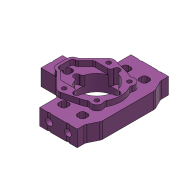
# Autodesk Inventor part: 16_030_TIBIA_SENSOR_BASE_R1
Saved by Autodesk Inventor 2021.2 (Build 252289000, 289)
## iProperties
Created: 2018-07-25
Part Number: 16_030_TIBIA_SENSOR_BASE_R1
Material: ABS プラスチック
Document SubType Name: Modeling
Designer: y6tada
Density: 1.06 g/cm^3
Appearance: 滑らか - 紫
Mass: 3.15209 g
Surface Area: 27.7865 cm^2
Volume: 2.97367 cm^3
Author: y6tada
Autodesk Inventor part; units mm, degrees
ref_plane "YZ Plane" through (0, 0, 0) normal (1, 0, 0) x (0, 1, 0)
ref_plane "XZ Plane" through (0, 0, 0) normal (0, 1, 0) x (-1, 0, 0)
ref_plane "作業平面1" through (0, 0, 0) normal (0, 0, 1) x (1, 0, 0)
sketch "スケッチ1" plane through (0, 0, 0) normal (0, 0, 1) x (1, 0, 0)
  line L0 (0, 0) -> (12.25, 0)
  line L1 (12.25, 0) -> (12.25, 14.0352) construction
  line L2 (-1.75, 17) -> (-1.75, 11.1093)
  line L3 (-2.0429, 10.4022) -> (-8.1522, 4.2929)
  line L4 (-8.8593, 4) -> (-14.25, 4)
  line L5 (-14.25, 4) -> (-14.25, 0.6)
  line L6 (-14.05, 0) -> (0, 0)
  line L7 (-8.7985, 4.3535) -> (-8.4451, 4) construction
  arc A0 (-8.8593, 4) -> (-8.1522, 4.2929) centre (-8.8593, 5) ccw
  arc A1 (-2.0429, 10.4022) -> (-1.75, 11.1093) centre (-2.75, 11.1093) ccw
  arc A2 (1.15, 17) -> (2.35, 17) centre (1.75, 17.8) ccw
  arc A3 (8.15, 17) -> (9.35, 17) centre (8.75, 17.8) ccw
  line L8 (12.25, 17) -> (9.35, 17)
  line L9 (8.15, 17) -> (2.35, 17)
  line L10 (1.15, 17) -> (-1.75, 17)
  line L11 (8.75, 17.8) -> (1.75, 17.8) construction
  arc A4 (-14.05, 0) -> (-14.25, 0.6) centre (-15.05, 0) ccw
  line L12 (12.455, 13.618) -> (14.045, 10.382)
  line L13 (14.25, 9.5) -> (14.25, 0)
  line L14 (14.25, 0) -> (12.25, 0)
  line L15 (12.25, 14.5) -> (12.25, 17)
  arc A5 (12.25, 14.5) -> (12.455, 13.618) centre (14.25, 14.5) ccw
  arc A6 (14.25, 9.5) -> (14.045, 10.382) centre (12.25, 9.5) ccw
  dimension "d5" = 1
  dimension "d9" = 1
  dimension "d21" = 14.25
  dimension "d22" = 4
  dimension "d23" = 8.8
  dimension "d24" = 45
  dimension "d26" = 17
  dimension "d27" = 0.8
  dimension "d28" = 1
  dimension "d29" = 3.5
  dimension "d30" = 3.5
  dimension "d31" = 1
  dimension "d32" = 0.8
  dimension "d73" = 1.75
  dimension "d74" = 14.25
  dimension "d76" = 14
  dimension "d77" = 2
  dimension "d78" = 2.5
  dimension "d79" = 5
  constraints: 32 end point, 14 point on circle, 8 tangent, 7 centre point, 6 horizontal, 5 point on line, 5 vertical, 3 perpendicular, 2 collinear, 2 equal radius, 1 coincident, 2 other
  measures "d5" radius of A0
  measures "d9" radius of A1
  measures "d21" distance from line of L5 point (0, 0)
  measures "d22" distance between parallel lines of L6 L4
  measures "d23" distance from line of L0.start L3
  measures "d24" angle of L3 L6
  measures "d26" distance of L0.end L8.start
  measures "d27" distance between parallel lines of L11 L9
  measures "d28" radius of A3
  measures "d29" distance from line of L11.start L1
  measures "d30" distance from line of L11.end L2
  measures "d31" radius of A4
  measures "d32" distance from line of L5 A4.centre
  measures "d73" distance from line of L0.start L2
  measures "d74" distance from line of L0.start L13
  measures "d76" distance between parallel lines of L2 L15
  measures "d77" radius of A5
  measures "d78" distance from line of A5.centre L8
  measures "d79" vertical distance of A6.centre A5.centre
extrude "押し出し1" add sketch "スケッチ1" along normal blind 6
sketch "スケッチ3" plane through (2.35, 17, 0) normal (0, 1, 0) x (1, 0, 0)
  circle A0 centre (-0.6, -3) radius 1.25
  circle A1 centre (6.4, -3) radius 1.25
  line L0 (6.4, -3) -> (-0.6, -3) construction
  line L1 (6.4, -3) -> (6.4, 0) construction
  line L2 (7, 0) -> (5.8, 0) construction
  line L3 (-0.6, -3) -> (-0.6, 0) construction
  line L4 (0, 0) -> (-1.2, 0) construction
  point P0 (-2.35, 0)
  dimension "d33" = 3
  dimension "d34" = 2.5
  constraints: 6 end point, 2 centre point, 2 midpoint, 2 vertical, 1 equal radius, 1 horizontal
  measures "d33" distance from line of point (-2.35, 0) L0
  measures "d34" diameter of A0
extrude "押し出し3" cut sketch "スケッチ3" against normal blind 5
mirror "ミラー2" about plane through (0, 0, 0) normal (0, -1, 0) of "押し出し1", "押し出し3"
sketch "スケッチ4" plane through (-14.25, -4, 0) normal (-1, 0, 0) x (0, 0, 1)
  circle A0 centre (3, 4) radius 1.25
  line L0 (0, 4) -> (3, 4) construction
  dimension "d37" = 3
  dimension "d38" = 2.5
  constraints: 2 end point, 1 centre point, 1 horizontal
  measures "d37" distance of L0.start L0.end
  measures "d38" diameter of A0
extrude "押し出し4" cut sketch "スケッチ4" against normal blind 5
sketch "スケッチ5" plane through (0, 0, 6) normal (0, 0, 1) x (1, 0, 0)
  circle A0 centre (2.5456, 0) radius 6.6
  line L0 (0, 0) -> (2.5456, 0) construction
  line L1 (-2.0429, 10.4022) -> (-8.1522, 4.2929) construction
  line L2 (0.7855, 7.5738) -> (-6.3238, 0.4645) construction
  dimension "d41" = 13.2
  dimension "d59" = 4
  constraints: 4 end point, 1 centre point, 1 coincident, 1 horizontal, 1 parallel, 1 tangent, 1 other
  measures "d41" diameter of A0
  measures "d59" distance between parallel lines of L2 L1
extrude "押し出し5" cut sketch "スケッチ5" against normal blind 8
sketch "スケッチ6" plane through (0, 0, 6) normal (0, 0, 1) x (1, 0, 0)
  line L0 (-4.9544, 0) -> (2.5456, 0) construction
  line L1 (-4.9544, 1.1) -> (-4.8334, 1.1)
  line L2 (-4.9544, -1.1) -> (-4.8334, -1.1)
  circle A0 centre (2.5456, 0) radius 6.6 construction
  arc A1 (-4.9544, 1.1) -> (-4.9544, -1.1) centre (-4.9544, 0) ccw
  arc A2 (-3.7793, -1.8857) -> (-4.8334, -1.1) centre (-4.8334, -2.2) ccw
  arc A3 (-4.8334, 1.1) -> (-3.7793, 1.8857) centre (-4.8334, 2.2) ccw
  arc A4 (-3.7793, 1.8857) -> (-3.7793, -1.8857) centre (2.5456, 0) ccw
  point P0 (-2.4621, -1.1)
  point P1 (-2.4621, 1.1)
  dimension "d76" = 14
  dimension "d44" = 7.5
  dimension "d47" = 1.1
  dimension "d53" = 1.1
  dimension "d55" = 1.1
  constraints: 8 point on circle, 6 end point, 6 tangent, 4 centre point, 3 horizontal, 2 concentric, 2 point on line, 1 coincident
  measures "d44" distance of L0.start L0.end
  measures "d47" radius of A1
  measures "d53" radius of A2
  measures "d55" radius of A3
extrude "押し出し6" cut sketch "スケッチ6" against normal blind 3.5
pattern_circular "円形状パターン1" count 4 over 360 about axis through (2.5456, 0, 6) along (0, 0, -1) of "押し出し6"
sketch "スケッチ9" plane through (0, 0, 6) normal (0, 0, 1) x (1, 0, 0)
  arc A0 (1.4456, -7.379) -> (0.6599, -6.3249) centre (0.3456, -7.379) ccw
  arc A1 (10.0456, -1.1) -> (11.1456, 0) centre (10.0456, 0) ccw
  line L0 (10.0456, -1.1) -> (9.9246, -1.1)
  arc A2 (9.9246, -1.1) -> (8.8705, -1.8857) centre (9.9246, -2.2) ccw
  arc A3 (4.4313, -6.3249) -> (8.8705, -1.8857) centre (2.5456, 0) ccw
  arc A4 (4.4313, -6.3249) -> (3.6456, -7.379) centre (4.7456, -7.379) ccw
  line L1 (3.6456, -7.379) -> (3.6456, -7.5)
  arc A5 (1.4456, -7.5) -> (3.6456, -7.5) centre (2.5456, -7.5) ccw
  line L2 (1.4456, -7.5) -> (1.4456, -7.379)
  arc A6 (10.4511, -4.3014) -> (11.5456, 0) centre (2.5456, 0) ccw
  arc A7 (7.7588, -7.883) -> (10.4286, -5.2133) centre (8.6267, -6.0811) ccw
  arc A8 (4.863, -8.6965) -> (6.847, -7.9056) centre (2.5456, 0) ccw
  arc A9 (10.4511, -4.3014) -> (10.4286, -5.2133) centre (11.3295, -4.7793) ccw
  arc A10 (7.7588, -7.883) -> (6.847, -7.9056) centre (7.3249, -8.784) ccw
  line L3 (-8.1522, -4.2929) -> (-2.7518, -9.6932)
  line L4 (-2.0429, -10.4022) -> (-8.1522, -4.2929) construction
  arc A11 (1.4456, -7.379) -> (0.6599, -6.3249) centre (0.3456, -7.379) ccw projected
  line L5 (-4.7518, -6.279) -> (-7.738, -3.2929)
  line L6 (-9.4544, -2) -> (-9.4544, 0)
  arc A12 (1.4456, -7.379) -> (0.3456, -6.279) centre (0.3456, -7.379) ccw
  line L7 (0.3456, -6.279) -> (-4.7518, -6.279)
  line L8 (2.5456, 0) -> (-9.4544, 0) construction
  line L9 (2.5456, 7.5) -> (2.5456, 0) construction
  line L10 (2.5456, 0) -> (10.0456, 0) construction
  line L11 (2.5456, 0) -> (2.5456, -7.5) construction
  line L12 (-2.0429, -10.4022) -> (-8.1522, -4.2929) construction
  circle A13 centre (2.5456, 0) radius 2.8146 construction
  arc A14 (-2.7518, -9.6932) -> (-0.8227, -10.2116) centre (-1.3376, -8.279) ccw
  line L13 (-0.8227, -10.2116) -> (4.863, -8.6965)
  line L14 (-10.4544, 0) -> (-9.4544, 0)
  line L15 (-10.4544, 0) -> (-10.4544, -2)
  line L16 (10.0456, 0) -> (11.1456, 0) construction
  line L17 (11.1456, 0) -> (11.5456, 0)
  line L18 (8.6267, -6.0811) -> (2.5456, 0) construction
  line L19 (-8.8593, -4) -> (-14.25, -4) construction
  arc A15 (-10.4544, -2) -> (-8.9846, -3.9284) centre (-8.4544, -2) ccw
  arc A16 (-8.1522, -4.2929) -> (-8.8593, -4) centre (-8.8593, -5) ccw construction
  arc A17 (-8.1522, -4.2929) -> (-8.5942, -4.0358) centre (-8.8593, -5) ccw
  line L20 (-8.4544, -3) -> (-8.4451, -3)
  arc A18 (-9.4544, -2) -> (-8.4544, -3) centre (-8.4544, -2) ccw
  arc A19 (-7.738, -3.2929) -> (-8.4451, -3) centre (-8.4451, -4) ccw
  line L21 (-8.9846, -3.9284) -> (-8.5942, -4.0358)
  point P0 (-10.4544, -1.5765)
  point P1 (-9.4544, -1.5765)
  point P2 (-10.05, -4)
  dimension "d80" = 1.1
  dimension "d84" = 7.5
  dimension "d86" = 1.1
  dimension "d87" = 1.1
  dimension "d91" = 2
  dimension "d92" = 2
  dimension "d93" = 12
  dimension "d94" = 9
  dimension "d95" = 2
  dimension "d96" = 8.6
  dimension "d97" = 45
  dimension "d98" = 1
  dimension "d113" = 1
  dimension "d114" = 1
  dimension "d115" = 1
  dimension "d116" = 1
  dimension "d117" = 1
  constraints: 38 end point, 32 point on circle, 23 centre point, 14 tangent, 5 point on line, 4 concentric, 4 horizontal, 4 vertical, 3 collinear, 2 equal radius, 2 perpendicular, 1 coincident, 1 parallel, 7 other
  measures "d80" radius of A0
  measures "d84" distance of L8.start L10.end
  measures "d86" radius of A5
  measures "d87" radius of A4
  measures "d91" radius of A14
  measures "d92" distance from line of L7 A14.centre
  measures "d93" distance between parallel lines of L11 L6
  measures "d94" radius of A8
  measures "d95" radius of A7
  measures "d96" distance of L18.start L18.end
  measures "d97" angle of L8 L18
  measures "d98" radius of A10
  measures "d113" distance between parallel lines of L15 L6
  measures "d114" distance between parallel lines of L3 L5
  measures "d115" radius of A18
  measures "d116" radius of A19
  measures "d117" distance between parallel lines of L19 L20
extrude "押し出し7" add sketch "スケッチ9" along normal blind 2
mirror "ミラー3" about plane through (0, 0, 0) normal (0, 1, 0) of "押し出し7"
fillet "フィレット1" radius 1 2 edges at (-4.7518, -6.279, 7) (-4.7518, 6.279, 7)
sketch "スケッチ10" plane through (0, 0, 6) normal (0, 0, 1) x (1, 0, 0)
  line L0 (-9.4544, -2) -> (-9.4544, 2) construction
  line L1 (-8.4544, 1.5) -> (-7.9544, 1.5)
  line L2 (-6.9544, 0.5) -> (-6.9544, -0.5)
  line L3 (-7.9544, -1.5) -> (-8.4544, -1.5)
  line L4 (-9.4544, -0.5) -> (-9.4544, 0.5)
  arc A0 (-8.4544, 1.5) -> (-9.4544, 0.5) centre (-8.4544, 0.5) ccw
  arc A1 (-6.9544, 0.5) -> (-7.9544, 1.5) centre (-7.9544, 0.5) ccw
  arc A2 (-7.9544, -1.5) -> (-6.9544, -0.5) centre (-7.9544, -0.5) ccw
  arc A3 (-9.4544, -0.5) -> (-8.4544, -1.5) centre (-8.4544, -0.5) ccw
  line L5 (-0.0673, 0) -> (5.25, 0) construction
  line L6 (1.25, -10) -> (2.25, -10)
  line L7 (3.25, -11) -> (3.25, -12)
  line L8 (2.25, -13) -> (1.25, -13)
  line L9 (0.25, -12) -> (0.25, -11)
  arc A4 (1.25, -10) -> (0.25, -11) centre (1.25, -11) ccw
  arc A5 (3.25, -11) -> (2.25, -10) centre (2.25, -11) ccw
  arc A6 (2.25, -13) -> (3.25, -12) centre (2.25, -12) ccw
  arc A7 (0.25, -12) -> (1.25, -13) centre (1.25, -12) ccw
  arc A8 (2.35, -17) -> (1.15, -17) centre (1.75, -17.8) ccw construction
  arc A9 (9.35, -17) -> (8.15, -17) centre (8.75, -17.8) ccw construction
  line L10 (1.75, -17.8) -> (8.75, -17.8) construction
  line L11 (5.25, -17.8) -> (5.25, -9.3652) construction
  line L12 (1.75, -13) -> (1.75, -10) construction
  line L13 (8.15, -17) -> (2.35, -17) projected
  line L14 (9.25, -10) -> (8.25, -10)
  line L15 (7.25, -11) -> (7.25, -12)
  line L16 (8.25, -13) -> (9.25, -13)
  line L17 (10.25, -12) -> (10.25, -11)
  arc A10 (10.25, -11) -> (9.25, -10) centre (9.25, -11) ccw
  arc A11 (8.25, -10) -> (7.25, -11) centre (8.25, -11) ccw
  arc A12 (7.25, -12) -> (8.25, -13) centre (8.25, -12) ccw
  arc A13 (9.25, -13) -> (10.25, -12) centre (9.25, -12) ccw
  line L18 (8.75, -13) -> (8.75, -10) construction
  line L19 (1.25, 10) -> (2.25, 10)
  line L20 (3.25, 11) -> (3.25, 12)
  line L21 (2.25, 13) -> (1.25, 13)
  line L22 (0.25, 12) -> (0.25, 11)
  arc A14 (0.25, 11) -> (1.25, 10) centre (1.25, 11) ccw
  arc A15 (2.25, 10) -> (3.25, 11) centre (2.25, 11) ccw
  arc A16 (3.25, 12) -> (2.25, 13) centre (2.25, 12) ccw
  arc A17 (1.25, 13) -> (0.25, 12) centre (1.25, 12) ccw
  line L23 (1.75, 13) -> (1.75, 10) construction
  line L24 (9.25, 10) -> (8.25, 10)
  arc A18 (9.25, 10) -> (10.25, 11) centre (9.25, 11) ccw
  line L25 (10.25, 12) -> (10.25, 11)
  arc A19 (7.25, 11) -> (8.25, 10) centre (8.25, 11) ccw
  arc A20 (10.25, 12) -> (9.25, 13) centre (9.25, 12) ccw
  line L26 (7.25, 11) -> (7.25, 12)
  line L27 (8.75, 13) -> (8.75, 10) construction
  line L28 (8.25, 13) -> (9.25, 13)
  arc A21 (8.25, 13) -> (7.25, 12) centre (8.25, 12) ccw
  line L29 (-9.4544, 2) -> (-9.4544, -2) projected
  point P0 (0, 0)
  dimension "d103" = 1
  dimension "d104" = 2.5
  dimension "d105" = 1
  dimension "d106" = 1
  dimension "d107" = 3
  dimension "d108" = 3
  dimension "d109" = 4
  dimension "d118" = 1
  constraints: 54 end point, 42 symmetric about line, 40 point on circle, 20 centre point, 16 tangent, 5 equal radius, 4 horizontal, 4 parallel, 3 midpoint, 2 perpendicular, 2 point on line, 1 collinear, 1 vertical, 14 other
  measures "d103" radius of A0
  measures "d104" distance between parallel lines of L0 L2
  measures "d105" radius of A4
  measures "d106" radius of A5
  measures "d107" distance between parallel lines of L7 L9
  measures "d108" distance between parallel lines of L8 L6
  measures "d109" distance between parallel lines of L13 L8
  measures "d118" distance of A1.centre A2.centre
extrude "押し出し8" cut sketch "スケッチ10" against normal blind 6
sketch "スケッチ11" plane through (0, 0, 8) normal (0, 0, 1) x (1, 0, 0)
  arc A0 (-0.8227, 10.2116) -> (-2.7518, 9.6932) centre (-1.3376, 8.279) ccw projected
  circle A1 centre (-1.3376, 8.279) radius 0.8
  circle A2 centre (8.6267, 6.0811) radius 0.8
  circle A3 centre (8.6267, -6.0811) radius 0.8
  circle A4 centre (-1.3376, -8.279) radius 0.8
  arc A5 (-0.8227, 10.2116) -> (-2.7518, 9.6932) centre (-1.3376, 8.279) ccw projected
  arc A6 (10.4286, 5.2133) -> (7.7588, 7.883) centre (8.6267, 6.0811) ccw projected
  arc A7 (7.7588, -7.883) -> (10.4286, -5.2133) centre (8.6267, -6.0811) ccw projected
  arc A8 (-2.7518, -9.6932) -> (-0.8227, -10.2116) centre (-1.3376, -8.279) ccw projected
  point P0 (0, 0)
  dimension "d119" = 1.6
  constraints: 4 centre point, 4 concentric, 3 equal radius, 1 coincident
  measures "d119" diameter of A1
extrude "押し出し9" cut sketch "スケッチ11" against normal blind 8
sketch "スケッチ12" plane through (0, 0, 8) normal (0, 0, 1) x (1, 0, 0)
  circle A0 centre (8.6267, -6.0811) radius 0.8 projected
  circle A1 centre (-1.3376, 8.279) radius 0.8 projected
  circle A2 centre (8.6267, 6.0811) radius 0.8 projected
  circle A3 centre (-1.3376, -8.279) radius 0.8 projected
  arc A4 (10.0456, -1.1) -> (10.0456, 1.1) centre (10.0456, 0) ccw projected
  line L0 (10.0456, -1.1) -> (9.9246, -1.1) projected
  arc A5 (9.9246, -1.1) -> (8.8705, -1.8857) centre (9.9246, -2.2) ccw projected
  arc A6 (4.4313, -6.3249) -> (8.8705, -1.8857) centre (2.5456, 0) ccw projected
  arc A7 (4.4313, -6.3249) -> (3.6456, -7.379) centre (4.7456, -7.379) ccw projected
  line L1 (3.6456, -7.379) -> (3.6456, -7.5) projected
  arc A8 (1.4456, -7.5) -> (3.6456, -7.5) centre (2.5456, -7.5) ccw projected
  line L2 (1.4456, -7.5) -> (1.4456, -7.379) projected
  arc A9 (1.4456, -7.379) -> (0.3456, -6.279) centre (0.3456, -7.379) ccw projected
  line L3 (0.3456, -6.279) -> (-4.3376, -6.279) projected
  arc A10 (-5.0447, -5.9861) -> (-4.3376, -6.279) centre (-4.3376, -5.279) ccw projected
  line L4 (-5.0447, -5.9861) -> (-7.738, -3.2929) projected
  arc A11 (-7.738, -3.2929) -> (-8.4451, -3) centre (-8.4451, -4) ccw projected
  line L5 (-8.4451, -3) -> (-8.4544, -3) projected
  arc A12 (-9.4544, -2) -> (-8.4544, -3) centre (-8.4544, -2) ccw projected
  line L6 (-9.4544, -2) -> (-9.4544, 2) projected
  arc A13 (-8.4544, 3) -> (-9.4544, 2) centre (-8.4544, 2) ccw projected
  line L7 (-8.4451, 3) -> (-8.4544, 3) projected
  arc A14 (-8.4451, 3) -> (-7.738, 3.2929) centre (-8.4451, 4) ccw projected
  line L8 (-5.0447, 5.9861) -> (-7.738, 3.2929) projected
  arc A15 (-4.3376, 6.279) -> (-5.0447, 5.9861) centre (-4.3376, 5.279) ccw projected
  line L9 (0.3456, 6.279) -> (-4.3376, 6.279) projected
  arc A16 (0.3456, 6.279) -> (1.4456, 7.379) centre (0.3456, 7.379) ccw projected
  line L10 (1.4456, 7.5) -> (1.4456, 7.379) projected
  arc A17 (3.6456, 7.5) -> (1.4456, 7.5) centre (2.5456, 7.5) ccw projected
  line L11 (3.6456, 7.379) -> (3.6456, 7.5) projected
  arc A18 (3.6456, 7.379) -> (4.4313, 6.3249) centre (4.7456, 7.379) ccw projected
  arc A19 (8.8705, 1.8857) -> (4.4313, 6.3249) centre (2.5456, 0) ccw projected
  arc A20 (8.8705, 1.8857) -> (9.9246, 1.1) centre (9.9246, 2.2) ccw projected
  line L12 (10.0456, 1.1) -> (9.9246, 1.1) projected
  arc A21 (10.4511, -4.3014) -> (10.4511, 4.3014) centre (2.5456, 0) ccw projected
  arc A22 (10.4286, 5.2133) -> (10.4511, 4.3014) centre (11.3295, 4.7793) ccw projected
  arc A23 (10.4286, 5.2133) -> (7.7588, 7.883) centre (8.6267, 6.0811) ccw projected
  arc A24 (6.847, 7.9056) -> (7.7588, 7.883) centre (7.3249, 8.784) ccw projected
  arc A25 (6.847, 7.9056) -> (4.863, 8.6965) centre (2.5456, 0) ccw projected
  line L13 (-0.8227, 10.2116) -> (4.863, 8.6965) projected
  arc A26 (-0.8227, 10.2116) -> (-2.7518, 9.6932) centre (-1.3376, 8.279) ccw projected
  line L14 (-8.1522, 4.2929) -> (-2.7518, 9.6932) projected
  arc A27 (-8.5942, 4.0358) -> (-8.1522, 4.2929) centre (-8.8593, 5) ccw projected
  line L15 (-8.9846, 3.9284) -> (-8.5942, 4.0358) projected
  arc A28 (-8.9846, 3.9284) -> (-10.4544, 2) centre (-8.4544, 2) ccw projected
  line L16 (-10.4544, -2) -> (-10.4544, 2) projected
  arc A29 (-10.4544, -2) -> (-8.9846, -3.9284) centre (-8.4544, -2) ccw projected
  line L17 (-8.9846, -3.9284) -> (-8.5942, -4.0358) projected
  arc A30 (-8.1522, -4.2929) -> (-8.5942, -4.0358) centre (-8.8593, -5) ccw projected
  line L18 (-8.1522, -4.2929) -> (-2.7518, -9.6932) projected
  arc A31 (-2.7518, -9.6932) -> (-0.8227, -10.2116) centre (-1.3376, -8.279) ccw projected
  line L19 (-0.8227, -10.2116) -> (4.863, -8.6965) projected
  arc A32 (4.863, -8.6965) -> (6.847, -7.9056) centre (2.5456, 0) ccw projected
  arc A33 (7.7588, -7.883) -> (6.847, -7.9056) centre (7.3249, -8.784) ccw projected
  arc A34 (7.7588, -7.883) -> (10.4286, -5.2133) centre (8.6267, -6.0811) ccw projected
  arc A35 (10.4511, -4.3014) -> (10.4286, -5.2133) centre (11.3295, -4.7793) ccw projected
  line L20 (-4.9544, 1.1) -> (-4.8334, 1.1) projected
  arc A36 (-4.9544, 1.1) -> (-4.9544, -1.1) centre (-4.9544, 0) ccw projected
  line L21 (-4.8334, -1.1) -> (-4.9544, -1.1) projected
  arc A37 (-3.7793, -1.8857) -> (-4.8334, -1.1) centre (-4.8334, -2.2) ccw projected
  arc A38 (-3.7793, 1.8857) -> (-3.7793, -1.8857) centre (2.5456, 0) ccw projected
  arc A39 (-4.8334, 1.1) -> (-3.7793, 1.8857) centre (-4.8334, 2.2) ccw projected
  arc A40 (0.6599, 6.3249) -> (-3.7793, 1.8857) centre (2.5456, 0) ccw projected
  arc A41 (-3.7793, -1.8857) -> (0.6599, -6.3249) centre (2.5456, 0) ccw projected
  arc A42 (-9.4544, -0.5) -> (-8.4544, -1.5) centre (-8.4544, -0.5) ccw projected
  line L22 (-9.4544, -0.5) -> (-9.4544, -2) projected
  arc A43 (-9.4544, -2) -> (-8.4544, -3) centre (-8.4544, -2) ccw projected
  line L23 (-8.4544, -3) -> (-8.4451, -3) projected
  arc A44 (-7.738, -3.2929) -> (-8.4451, -3) centre (-8.4451, -4) ccw projected
  line L24 (-7.738, -3.2929) -> (-5.0447, -5.9861) projected
  arc A45 (-5.0447, -5.9861) -> (-4.3376, -6.279) centre (-4.3376, -5.279) ccw projected
  line L25 (-4.3376, -6.279) -> (0.3456, -6.279) projected
  arc A46 (0.6599, -6.3249) -> (0.3456, -6.279) centre (0.3456, -7.379) ccw projected
  arc A47 (-3.7793, -1.8857) -> (0.6599, -6.3249) centre (2.5456, 0) ccw projected
  arc A48 (-3.7793, -1.8857) -> (-4.8334, -1.1) centre (-4.8334, -2.2) ccw projected
  line L26 (-4.8334, -1.1) -> (-4.9544, -1.1) projected
  arc A49 (-4.9544, 1.1) -> (-4.9544, -1.1) centre (-4.9544, 0) ccw projected
  line L27 (-4.9544, 1.1) -> (-4.8334, 1.1) projected
  arc A50 (-4.8334, 1.1) -> (-3.7793, 1.8857) centre (-4.8334, 2.2) ccw projected
  arc A51 (0.6599, 6.3249) -> (-3.7793, 1.8857) centre (2.5456, 0) ccw projected
  arc A52 (0.3456, 6.279) -> (0.6599, 6.3249) centre (0.3456, 7.379) ccw projected
  line L28 (0.3456, 6.279) -> (-4.3376, 6.279) projected
  arc A53 (-4.3376, 6.279) -> (-5.0447, 5.9861) centre (-4.3376, 5.279) ccw projected
  line L29 (-5.0447, 5.9861) -> (-7.738, 3.2929) projected
  arc A54 (-8.4451, 3) -> (-7.738, 3.2929) centre (-8.4451, 4) ccw projected
  line L30 (-8.4451, 3) -> (-8.4544, 3) projected
  arc A55 (-8.4544, 3) -> (-9.4544, 2) centre (-8.4544, 2) ccw projected
  line L31 (-9.4544, 2) -> (-9.4544, 0.5) projected
  arc A56 (-8.4544, 1.5) -> (-9.4544, 0.5) centre (-8.4544, 0.5) ccw projected
  line L32 (-8.4544, 1.5) -> (-7.9544, 1.5) projected
  arc A57 (-6.9544, 0.5) -> (-7.9544, 1.5) centre (-7.9544, 0.5) ccw projected
  line L33 (-6.9544, 0.5) -> (-6.9544, -0.5) projected
  arc A58 (-7.9544, -1.5) -> (-6.9544, -0.5) centre (-7.9544, -0.5) ccw projected
  line L34 (-7.9544, -1.5) -> (-8.4544, -1.5) projected
  line L35 (-8.9846, 3.9284) -> (-8.5942, 4.0358) projected
  arc A59 (-8.8593, 4) -> (-8.5942, 4.0358) centre (-8.8593, 5) ccw projected
  line L36 (-8.8593, 4) -> (-14.25, 4) projected
  line L37 (-14.25, 4) -> (-14.25, 0.6) projected
  arc A60 (-14.25, -0.6) -> (-14.25, 0.6) centre (-15.05, 0) ccw projected
  line L38 (-14.25, -4) -> (-14.25, -0.6) projected
  line L39 (-8.8593, -4) -> (-14.25, -4) projected
  arc A61 (-8.5942, -4.0358) -> (-8.8593, -4) centre (-8.8593, -5) ccw projected
  line L40 (-8.5942, -4.0358) -> (-8.9846, -3.9284) projected
  arc A62 (-10.4544, -2) -> (-8.9846, -3.9284) centre (-8.4544, -2) ccw projected
  line L41 (-10.4544, -2) -> (-10.4544, 2) projected
  arc A63 (-8.9846, 3.9284) -> (-10.4544, 2) centre (-8.4544, 2) ccw projected
  arc A64 (2.25, 10) -> (3.25, 11) centre (2.25, 11) ccw projected
  line L42 (2.25, 10) -> (1.25, 10) projected
  arc A65 (0.25, 11) -> (1.25, 10) centre (1.25, 11) ccw projected
  line L43 (0.25, 11) -> (0.25, 12) projected
  arc A66 (1.25, 13) -> (0.25, 12) centre (1.25, 12) ccw projected
  line L44 (1.25, 13) -> (2.25, 13) projected
  arc A67 (3.25, 12) -> (2.25, 13) centre (2.25, 12) ccw projected
  line L45 (3.25, 12) -> (3.25, 11) projected
  arc A68 (8.25, -10) -> (7.25, -11) centre (8.25, -11) ccw projected
  line L46 (8.25, -10) -> (9.25, -10) projected
  arc A69 (10.25, -11) -> (9.25, -10) centre (9.25, -11) ccw projected
  line L47 (10.25, -11) -> (10.25, -12) projected
  arc A70 (9.25, -13) -> (10.25, -12) centre (9.25, -12) ccw projected
  line L48 (9.25, -13) -> (8.25, -13) projected
  arc A71 (7.25, -12) -> (8.25, -13) centre (8.25, -12) ccw projected
  line L49 (7.25, -12) -> (7.25, -11) projected
  arc A72 (1.25, -10) -> (0.25, -11) centre (1.25, -11) ccw projected
  line L50 (1.25, -10) -> (2.25, -10) projected
  arc A73 (3.25, -11) -> (2.25, -10) centre (2.25, -11) ccw projected
  line L51 (3.25, -11) -> (3.25, -12) projected
  arc A74 (2.25, -13) -> (3.25, -12) centre (2.25, -12) ccw projected
  line L52 (2.25, -13) -> (1.25, -13) projected
  arc A75 (0.25, -12) -> (1.25, -13) centre (1.25, -12) ccw projected
  line L53 (0.25, -12) -> (0.25, -11) projected
  arc A76 (7.25, 11) -> (8.25, 10) centre (8.25, 11) ccw projected
  line L54 (7.25, 11) -> (7.25, 12) projected
  arc A77 (8.25, 13) -> (7.25, 12) centre (8.25, 12) ccw projected
  line L55 (8.25, 13) -> (9.25, 13) projected
  arc A78 (10.25, 12) -> (9.25, 13) centre (9.25, 12) ccw projected
  line L56 (10.25, 12) -> (10.25, 11) projected
  arc A79 (9.25, 10) -> (10.25, 11) centre (9.25, 11) ccw projected
  line L57 (9.25, 10) -> (8.25, 10) projected
  arc A80 (10.4511, -4.3014) -> (10.4511, 4.3014) centre (2.5456, 0) ccw projected
  arc A81 (10.4511, -4.3014) -> (10.4286, -5.2133) centre (11.3295, -4.7793) ccw projected
  arc A82 (7.7588, -7.883) -> (10.4286, -5.2133) centre (8.6267, -6.0811) ccw projected
  arc A83 (7.7588, -7.883) -> (6.847, -7.9056) centre (7.3249, -8.784) ccw projected
  arc A84 (4.863, -8.6965) -> (6.847, -7.9056) centre (2.5456, 0) ccw projected
  line L58 (4.863, -8.6965) -> (-0.8227, -10.2116) projected
  arc A85 (-2.7518, -9.6932) -> (-0.8227, -10.2116) centre (-1.3376, -8.279) ccw projected
  line L59 (-2.0429, -10.4022) -> (-2.7518, -9.6932) projected
  arc A86 (-1.75, -11.1093) -> (-2.0429, -10.4022) centre (-2.75, -11.1093) ccw projected
  line L60 (-1.75, -17) -> (-1.75, -11.1093) projected
  line L61 (1.15, -17) -> (-1.75, -17) projected
  arc A87 (2.35, -17) -> (1.15, -17) centre (1.75, -17.8) ccw projected
  line L62 (8.15, -17) -> (2.35, -17) projected
  arc A88 (9.35, -17) -> (8.15, -17) centre (8.75, -17.8) ccw projected
  line L63 (12.25, -17) -> (9.35, -17) projected
  line L64 (12.25, -14.5) -> (12.25, -17) projected
  arc A89 (12.455, -13.618) -> (12.25, -14.5) centre (14.25, -14.5) ccw projected
  line L65 (14.045, -10.382) -> (12.455, -13.618) projected
  arc A90 (14.045, -10.382) -> (14.25, -9.5) centre (12.25, -9.5) ccw projected
  line L66 (14.25, 9.5) -> (14.25, -9.5) projected
  arc A91 (14.25, 9.5) -> (14.045, 10.382) centre (12.25, 9.5) ccw projected
  line L67 (14.045, 10.382) -> (12.455, 13.618) projected
  arc A92 (12.25, 14.5) -> (12.455, 13.618) centre (14.25, 14.5) ccw projected
  line L68 (12.25, 14.5) -> (12.25, 17) projected
  line L69 (12.25, 17) -> (9.35, 17) projected
  arc A93 (8.15, 17) -> (9.35, 17) centre (8.75, 17.8) ccw projected
  line L70 (8.15, 17) -> (2.35, 17) projected
  arc A94 (1.15, 17) -> (2.35, 17) centre (1.75, 17.8) ccw projected
  line L71 (1.15, 17) -> (-1.75, 17) projected
  line L72 (-1.75, 17) -> (-1.75, 11.1093) projected
  arc A95 (-2.0429, 10.4022) -> (-1.75, 11.1093) centre (-2.75, 11.1093) ccw projected
  line L73 (-2.0429, 10.4022) -> (-2.7518, 9.6932) projected
  arc A96 (-0.8227, 10.2116) -> (-2.7518, 9.6932) centre (-1.3376, 8.279) ccw projected
  line L74 (-0.8227, 10.2116) -> (4.863, 8.6965) projected
  arc A97 (6.847, 7.9056) -> (4.863, 8.6965) centre (2.5456, 0) ccw projected
  arc A98 (6.847, 7.9056) -> (7.7588, 7.883) centre (7.3249, 8.784) ccw projected
  arc A99 (10.4286, 5.2133) -> (7.7588, 7.883) centre (8.6267, 6.0811) ccw projected
  arc A100 (10.4286, 5.2133) -> (10.4511, 4.3014) centre (11.3295, 4.7793) ccw projected
  point P0 (0, 0)
